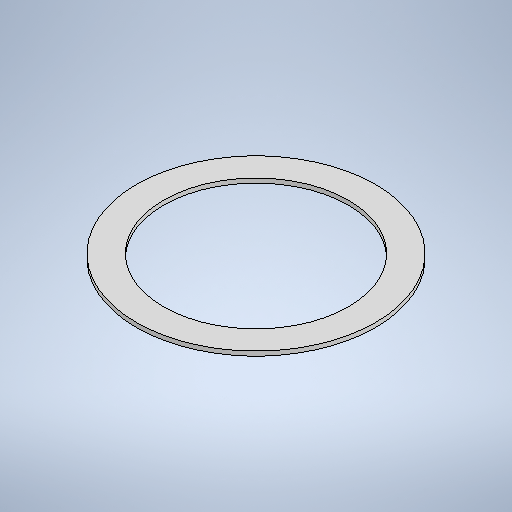
# Autodesk Inventor part: DSB 114 lap joint flange
Saved by Autodesk Inventor 2025.1 (Build 291241020, 241B)
## iProperties
Created: 2024-12-09
Part Number: DSB 114 lap joint flange
Material: Stainless Steel
Document SubType Name: Sheet Metal
Designer: user
Mass: 1674.72 g
Surface Area: 927.524 cm^2
Volume: 209.34 cm^3
Density: 8 g/cm^3
Flat Pattern Width: 21.8 cm
Flat Pattern Length: 21.8 cm
Flat Pattern Area: 475.24 cm^2
Sheet Metal Rule: AISI304 4mm Die 32
Sheet Metal Width: 218.000 mm
Sheet Metal Length: 218.000 mm
Sheet Metal Area: 47524.000 mm^2
Appearance: Default
Octaeder_side: 55.919 mm
Octaeder_flange_lenth: 72.500 mm
Author: user
Autodesk Inventor part; units mm, degrees
ref_plane "YZ Plane" through (0, 0, 0) normal (1, 0, 0) x (0, 1, 0)
ref_plane "XZ Plane" through (0, 0, 0) normal (0, 1, 0) x (-1, 0, 0)
ref_plane "XY Plane" through (0, 0, 0) normal (0, 0, 1) x (1, 0, 0)
sketch "Sketch1" plane through (0, 0, 0) normal (0, 0, 1) x (1, 0, 0)
  circle A0 centre (0, 0) radius 84.25
  circle A1 centre (0, 0) radius 109
  line L0 (77.0746, -77.0746) -> (-77.0746, 77.0746) construction
  line L1 (-77.0746, -77.0746) -> (77.0746, 77.0746) construction
  point P0 (0, 84.25)
  dimension "d44" = 168.5
  dimension "d23" = 218
  dimension "d45" = 24.75
  measures "d23" diameter of A1
extrude "Plate1" add sketch "Sketch1" along normal blind 4
equation "\"d2\" = Thickness"
equation "\"BendReliefWidth\" = Thickness"
equation "\"BendReliefDepth\" = 0.5 * Thickness"
equation "\"CornerReliefSize\" = 4 * Thickness"
equation "\"MinimumRemnant\" = 2 * Thickness"
equation "\"TransitionRadius\" = BendRadius"
equation "\"JacobiRadiusSize\" = BendRadius"
equation "\"GapSize\" = Thickness"
equation "\"Octaeder_side\" = d41"
equation "\"Octaeder_flange_lenth\" = d42"
equation "\"Thickness\" = 4"
equation "\"BendRadius\" = 6"
equation "\"d41\" = 55.918831"
equation "\"d42\" = 72.5"
body "Solid1"
